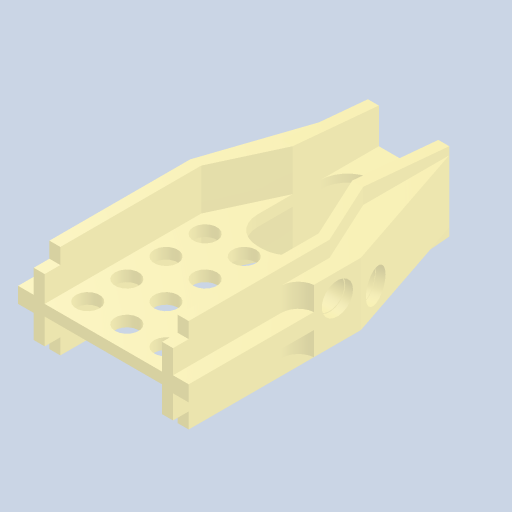
# Autodesk Inventor part: ProbeMount_vC
Saved by Autodesk Inventor 2023 (Build 270158000, 158)
## iProperties
Created: 2021-05-04
Part Number: ProbeMount_vC
Material: Nylon 6/6
Document SubType Name: Modeling
Designer: Pip
Density: 1.13 g/cm^3
Appearance: Snow
Mass: 0.321763 g
Surface Area: 8.04977 cm^2
Volume: 0.284746 cm^3
InterProbeDist: 2.000 mm
WallThickness: 0.700 mm
Author: Pip
Autodesk Inventor part; units mm, degrees
ref_plane "YZ Plane" through (0, 0, 0) normal (1, 0, 0) x (0, 1, 0)
ref_plane "XZ Plane" through (0, 0, 0) normal (0, 1, 0) x (-1, 0, 0)
ref_plane "XY Plane" through (0, 0, 0) normal (0, 0, 1) x (1, 0, 0)
sketch "Sk:Base" plane through (0, 0, 0) normal (0, 1, 0) x (-1, 0, 0)
  line L0 (0, -5) -> (-3.75, -5)
  line L1 (-3.75, -5) -> (-3.75, 5)
  line L2 (-3.75, 5) -> (0, 5)
  line L3 (0, 5) -> (0, -5)
  line L4 (-3.75, -5) -> (-1.9, -9)
  line L5 (-1.9, -9) -> (0, -9)
  line L6 (0, -9) -> (0, -5)
  line L7 (-3.75, 5) -> (-4.45, 5)
  line L8 (-4.45, -5) -> (-3.75, -5)
  line L9 (-3.75, -5) -> (-3.75, 5)
  line L10 (-2.6, -9) -> (-1.9, -9)
  line L11 (0, 5) -> (-2.5, 5)
  line L12 (-4.45, -5) -> (-4.45, 5)
  line L13 (-4.45, -5) -> (-2.6, -9)
  line L14 (-1.9, -9) -> (-1.9, -5)
  line L15 (-5.45, -3) -> (-4.45, -3)
  line L16 (-5.45, -3) -> (-5.45, -6)
  line L17 (-4.45, 5) -> (-5.45, 5)
  line L18 (-5.45, 5) -> (-5.45, -3)
  line L19 (-5.45, -3) -> (-4.45, -3)
  line L20 (-4.45, -3) -> (-4.45, 5)
  line L21 (-2.6, -9) -> (-1.9, -9)
  line L22 (-1.9, -9) -> (-1.9, -14.5)
  line L23 (-1.9, -14.5) -> (-2.6, -14.5)
  line L24 (-2.6, -14.5) -> (-2.6, -9)
  line L25 (-1.9, -14.5) -> (0, -14.5)
  line L26 (0, -14.5) -> (0, -12.5)
  line L27 (0, -12.5) -> (-1.9, -12.5)
  line L28 (-1.9, -12.5) -> (-1.9, -14.5)
  line L29 (-2.6, -14.5) -> (-5.45, -6)
  point P0 (0, 0)
  dimension "d4" = 3.75
  dimension "d3" = 10
  dimension "d5" = 0
  dimension "d6" = 1.9
  dimension "d7" = 0
  dimension "d1" = 0.7
  dimension "d40" = 5
  dimension "d41" = 4
  dimension "d129" = 3
  dimension "d148" = 8
  dimension "d167" = 5.5
  dimension "d168" = 0.7
  dimension "d169" = 2
  dimension "d172" = 1
  dimension "d173" = 1
  dimension "d232" = 18.536
  dimension "d289" = 3.75
  constraints: 60 end point, 11 parallel, 8 horizontal, 5 perpendicular, 3 point on line, 3 vertical
  measures "d4" distance of L0.start L0.end
  measures "d3" distance of L0.end L1.end
  measures "d5" distance from line of point (0, 0) L3
  measures "d6" distance of L4.end L5.end
  measures "d7" horizontal distance of L0.start L5.end
  measures "d1" distance between parallel lines of L12 L1
  measures "d40" distance from line of point (0, 0) L2
  measures "d41" distance between parallel lines of L0 L5
  measures "d129" distance of L15.start L16.end
  measures "d148" distance of L17.end L18.end
  measures "d167" distance of L21.end L22.end
  measures "d168" distance between parallel lines of L24 L22
  measures "d169" distance of L26.end L25.end
  measures "d172" distance between parallel lines of L12 L18
  measures "d173" distance between parallel lines of L12 L16
  measures "d232" angle of L24 L29
  measures "d289" distance between parallel lines of L1 L26
extrude "Ex:Midline" add sketch "Sk:Base" along normal blind 0.35 contours L0 L1 L2 L3 | L14 L4 L0
extrude "Ex:FrontSupport" add sketch "Sk:Base" along normal blind 0.25 contours L27 L26 L25 L22
extrude "Ex:SideRidge" add sketch "Sk:Base" along normal blind 0.5 contours L12 L15 L18 L17
extrude "Ex:SideWall" add sketch "Sk:Base" along normal blind 3 contours L8 L12 L7 L1 | L4 L10 L13 L8 | L22 L23 L24 L10
sketch "Sk:BaseHole" plane through (0, 0.35, 0) normal (0, 1, 0) x (1, 0, 0)
  circle A0 centre (2.5, -3.5) radius 0.75
  line L0 (0, -5) -> (3.75, -5) projected
  line L1 (0, 5) -> (0, -5) projected
  point P0 (0, 0)
  point P1 (0, 10)
  dimension "d68" = 1.5
  dimension "d69" = 1.5
  dimension "d79" = 2.5
  constraints: 1 centre point
  measures "d68" diameter of A0
  measures "d69" distance from line of A0.centre L0
  measures "d79" distance from line of A0.centre L1
extrude "Ex:BaseHole" cut sketch "Sk:BaseHole" against normal mid plane 5.3
pattern_linear "Pat:BaseHoles" count 4 spacing 2.5 along (0, 0, -1) count 2 spacing 2.5 along (-1, 0, 0) of "Ex:BaseHole"
fillet "Fillet:Support" radius 1.75 2 edges at (1.9, 0.175, -5) (1.9, 0.125, -12.5)
extrude "Ex:Widening" add sketch "Sk:Base" along normal blind 2 contours L22 L23 L24 L10 | L13 L24 L29 L16 L15 L12
fillet "Fillet:Side" radius 1.1 1 edges at (4.45, 1.25, -3)
sketch "Sk:FrontTaper" plane through (2.6, 3, -9) normal (1, 0, 0) x (0, 0, -1)
  line L0 (5.5, 0) -> (0, 0) projected
  line L1 (0, -1) -> (5.5, -1) projected
  line L2 (0, 0) -> (5.5, 0)
  line L3 (5.5, 0) -> (5.5, -1)
  line L4 (5.5, -1) -> (0, -1)
  line L5 (0, -1) -> (0, 0)
  line L6 (0, 0) -> (-4, 0) projected
  line L7 (0, 0) -> (5.5, -0.5)
  point P0 (-9, -3)
  point P1 (5.5, -0.5)
  point P2 (4.5, 0)
  dimension "d219" = 1
  dimension "d222" = 0.5
  dimension "d223" = 0
  constraints: 10 end point, 2 parallel, 1 horizontal, 1 perpendicular
  measures "d219" distance of L4.end L0.end
  measures "d222" distance of L0.start L7.end
  measures "d223" distance from line of L3 L7.end
extrude "Ex:FrontTaper" cut sketch "Sk:FrontTaper" against normal up to next contours L3 L7 L0
sketch "Sk:LidNotch" plane through (4.45, 0.5, 5) normal (1, 0, 0) x (0, 0, -1)
  line L0 (0, -0.15) -> (0, 2.5) projected
  line L1 (0, 2.5) -> (1, 2.5)
  line L2 (1, 2.5) -> (1, 1.5)
  line L3 (1, 1.5) -> (0, 1.5)
  line L4 (0, 1.5) -> (0, 2.5)
  line L5 (0, 2.5) -> (10, 2.5) projected
  point P0 (5, -0.5)
  point P1 (0, 1.5)
  dimension "d224" = 1
  dimension "d225" = 1
  constraints: 8 end point, 2 parallel, 1 horizontal, 1 perpendicular
  measures "d224" distance between parallel lines of L0 L2
  measures "d225" distance between parallel lines of L5 L3
extrude "Ex:LidNotch" cut sketch "Sk:LidNotch" against normal up to next
mirror "Mirror1" about plane through (0, 0, -5) normal (-1, 0, 0)
mirror "Mirror2" about plane through (0.95, 0, -13.5) normal (0, -1, 0)
sketch "Sk:ThreadHole1" plane through (5.45, 2, -3) normal (1, 0, 0) x (0, 0, -1)
  circle A0 centre (1.5, -1.5) radius 0.95
  circle A1 centre (1.5, -1.5) radius 1
  line L0 (0, 0) -> (3, 0) projected
  line L1 (0, -1.5) -> (0, 0) projected
  point P0 (-3, -2)
  dimension "d130" = 1.9
  dimension "d131" = 2
  dimension "d199" = 1.5
  dimension "d200" = 1.5
  constraints: 2 centre point, 1 concentric
  measures "d130" diameter of A0
  measures "d131" diameter of A1
  measures "d199" distance from line of L0 A0.centre
  measures "d200" distance from line of L1 A0.centre
sketch "Sk:ThreadHole2" plane through (4.4125, -2, -9.0944) normal (0.9481241, 0, -0.3179004) x (-0.3179004, 0, -0.9481241)
  circle A0 centre (-1.7637, 1.5) radius 1
  circle A1 centre (-1.7637, 1.5) radius 0.95
  line L0 (-3.2637, 0) -> (5.7014, 0) projected
  line L1 (-3.2637, 0) -> (-3.2637, 4) projected
  point P0 (-7.2199, 2)
  dimension "d134" = 1.9
  dimension "d135" = 2
  dimension "d217" = 1.5
  dimension "d228" = 1.5
  constraints: 2 centre point, 1 concentric
  measures "d134" diameter of A1
  measures "d135" diameter of A0
  measures "d217" distance from line of L0 A0.centre
  measures "d228" distance from line of L1 A0.centre
extrude "Ex:ThreadHole1" cut sketch "Sk:ThreadHole1" against normal blind 1.5 contours A0
extrude "Ex:ThreadEntry1" cut sketch "Sk:ThreadHole1" against normal blind 0.5 contours A0 | A1
extrude "Ex:ThreadHole2" cut sketch "Sk:ThreadHole2" against normal blind 1.5 contours A1
extrude "Ex:ThreadEntry2" cut sketch "Sk:ThreadHole2" against normal blind 0.5 contours A0 | A1
pattern_circular "Pat:Threads" count 2 over 360 about axis through (0, 0, -10) along (0, 0, 1) of "Ex:ThreadEntry1", "Ex:ThreadEntry2", "Ex:ThreadHole2", "Ex:ThreadHole1"
equation "\"d40\" = 0.5 * d3"
body "Solid1"
